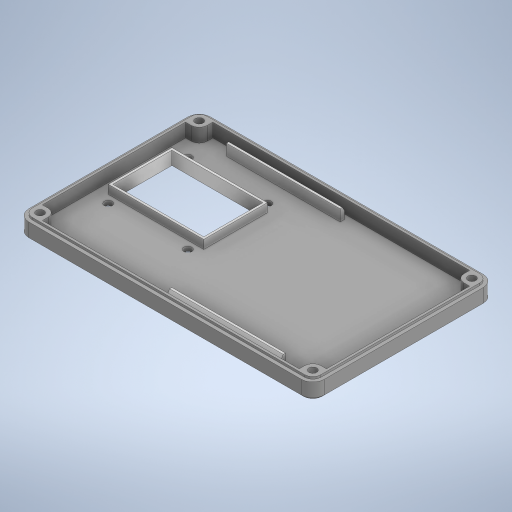
# Autodesk Inventor part: housing_top
Saved by Autodesk Inventor 2023 (Build 270158000, 158)
## iProperties
Created: 2023-05-16
Part Number: housing_top
Material: Generic
Document SubType Name: Modeling
Designer: mark
Density: 1 g/cm^3
Appearance: Default
Author: mark
Autodesk Inventor part; units mm, degrees
ref_plane "YZ Plane" through (0, 0, 0) normal (1, 0, 0) x (0, 1, 0)
ref_plane "XZ Plane" through (0, 0, 0) normal (0, 1, 0) x (-1, 0, 0)
ref_plane "XY Plane" through (0, 0, 0) normal (0, 0, 1) x (1, 0, 0)
sketch "Sketch1" plane through (0, 0, 0) normal (0, 1, 0) x (-1, 0, 0)
  line L0 (59.6914, -40.823) -> (-60.3086, -40.823)
  line L1 (-65.3086, -35.823) -> (-65.3086, 34.177)
  line L2 (-60.3086, 39.177) -> (59.6914, 39.177)
  line L3 (64.6914, 34.177) -> (64.6914, -35.823)
  arc A0 (59.6914, -40.823) -> (64.6914, -35.823) centre (59.6914, -35.823) ccw
  arc A1 (-65.3086, -35.823) -> (-60.3086, -40.823) centre (-60.3086, -35.823) ccw
  arc A2 (64.6914, 34.177) -> (59.6914, 39.177) centre (59.6914, 34.177) ccw
  arc A3 (-60.3086, 39.177) -> (-65.3086, 34.177) centre (-60.3086, 34.177) ccw
  point P0 (0, 0)
  point P1 (64.6914, -40.823)
  point P2 (-65.3086, 39.177)
  point P3 (64.6914, 39.177)
  dimension "d0" = 80
  dimension "d1" = 130
  dimension "d2" = 5
  dimension "d3" = 5
  dimension "d4" = 5
  dimension "d5" = 5
  constraints: 8 end point, 8 point on circle, 8 tangent, 6 point on line, 4 centre point, 2 parallel, 1 horizontal, 1 perpendicular
  measures "d0" distance of point (64.691, 39.177) point (64.691, -40.823)
  measures "d1" distance of point (-65.309, 39.177) point (64.691, 39.177)
  measures "d2" radius of A0
  measures "d3" radius of A1
  measures "d4" radius of A2
  measures "d5" radius of A3
extrude "Extrusion1" add sketch "Sketch1" along normal blind 2
sketch "Sketch2" plane through (0, 2, 0) normal (0, 1, 0) x (1, 0, 0)
  line L0 (-64.6914, 35.823) -> (-64.6914, -34.177) projected
  line L1 (-64.6914, 35.823) -> (-64.6914, -34.177)
  arc A0 (-64.6914, -34.177) -> (-59.6914, -39.177) centre (-59.6914, -34.177) ccw projected
  arc A1 (-64.6914, -34.177) -> (-59.6914, -39.177) centre (-59.6914, -34.177) ccw
  arc A2 (-59.6914, 40.823) -> (-64.6914, 35.823) centre (-59.6914, 35.823) ccw
  arc A3 (65.3086, 35.823) -> (60.3086, 40.823) centre (60.3086, 35.823) ccw projected
  arc A4 (65.3086, 35.823) -> (60.3086, 40.823) centre (60.3086, 35.823) ccw
  line L2 (-62.1914, 35.823) -> (-62.1914, -34.177)
  line L3 (65.3086, -34.177) -> (65.3086, 35.823) projected
  line L4 (65.3086, 35.823) -> (65.3086, -34.177)
  arc A5 (60.3086, -39.177) -> (65.3086, -34.177) centre (60.3086, -34.177) ccw projected
  line L5 (-59.6914, -39.177) -> (60.3086, -39.177) projected
  line L6 (60.3086, -39.177) -> (-59.6914, -39.177)
  line L7 (60.3086, 40.823) -> (-59.6914, 40.823) projected
  line L8 (-59.6914, 40.823) -> (60.3086, 40.823)
  line L9 (62.8086, 35.823) -> (62.8086, -34.177)
  line L10 (60.3086, -36.677) -> (-59.6914, -36.677)
  line L11 (-59.6914, 38.323) -> (60.3086, 38.323)
  arc A6 (-59.6914, 38.323) -> (-62.1914, 35.823) centre (-59.6914, 35.823) ccw
  arc A7 (62.8086, 35.823) -> (60.3086, 38.323) centre (60.3086, 35.823) ccw
  arc A8 (60.3086, -36.677) -> (62.8086, -34.177) centre (60.3086, -34.177) ccw
  arc A9 (-62.1914, -34.177) -> (-59.6914, -36.677) centre (-59.6914, -34.177) ccw
  arc A10 (-59.6914, 39.323) -> (-63.1914, 35.823) centre (-59.6914, 35.823) ccw
  arc A11 (63.8086, 35.823) -> (60.3086, 39.323) centre (60.3086, 35.823) ccw
  arc A12 (60.3086, -37.677) -> (63.8086, -34.177) centre (60.3086, -34.177) ccw
  arc A13 (-63.1914, -34.177) -> (-59.6914, -37.677) centre (-59.6914, -34.177) ccw
  line L12 (-63.1914, 35.823) -> (-63.1914, -34.177)
  line L13 (-59.6914, -37.677) -> (60.3086, -37.677)
  line L14 (63.8086, -34.177) -> (63.8086, 35.823)
  line L15 (60.3086, 39.323) -> (-59.6914, 39.323)
  line L16 (-59.6914, 32.323) -> (-62.1914, 32.323)
  line L17 (-56.1914, 35.823) -> (-56.1914, 38.323)
  arc A14 (-59.6914, 32.323) -> (-56.1914, 35.823) centre (-59.6914, 35.823) ccw
  line L18 (0.3086, 40.823) -> (0.3086, 33.323)
  line L19 (65.3086, 0.823) -> (44.6486, 0.823)
  line L20 (60.3086, 32.323) -> (62.8086, 32.323)
  line L21 (56.8086, 35.823) -> (56.8086, 38.323)
  arc A15 (56.8086, 35.823) -> (60.3086, 32.323) centre (60.3086, 35.823) ccw
  line L22 (-59.6914, -30.677) -> (-62.1914, -30.677)
  line L23 (-56.1914, -34.177) -> (-56.1914, -36.677)
  arc A16 (-56.1914, -34.177) -> (-59.6914, -30.677) centre (-59.6914, -34.177) ccw
  line L24 (56.8086, -34.177) -> (56.8086, -36.677)
  arc A17 (60.3086, -30.677) -> (56.8086, -34.177) centre (60.3086, -34.177) ccw
  line L25 (60.3086, -30.677) -> (62.8086, -30.677)
  point P0 (0, 0)
  point P1 (60.3086, -34.2192)
  point P2 (65.3086, -34.2192)
  point P3 (59.6599, -39.177)
  point P4 (56.8086, 38.323)
  point P5 (62.8086, -30.677)
  point P6 (56.8086, -36.677)
  point P7 (-56.1914, -36.677)
  point P8 (-62.1914, -30.677)
  dimension "d51" = 5
  dimension "d8" = 2.5
  dimension "d9" = 2.5
  dimension "d10" = 2.5
  dimension "d11" = 2.5
  dimension "d12" = 7
  dimension "d13" = 7
  dimension "d14" = 7
  dimension "d15" = 7
  dimension "d34" = 3.5
  dimension "d50" = 2.5
  dimension "d52" = 5
  dimension "d53" = 2.5
  constraints: 44 end point, 30 point on circle, 17 symmetric about line, 15 centre point, 11 coincident, 10 point on line, 10 tangent, 6 equal length, 3 vertical, 2 horizontal, 2 midpoint, 2 perpendicular, 7 other
  measures "d8" distance between parallel lines of L0 L2
  measures "d9" distance between parallel lines of L7 L11
  measures "d10" distance between parallel lines of L3 L9
  measures "d11" distance between parallel lines of L5 L10
  measures "d12" diameter of A10
  measures "d13" diameter of A11
  measures "d14" diameter of A12
  measures "d15" diameter of A13
  measures "d34" radius of A17
  measures "d50" radius of A8
  measures "d52" radius of A4
  measures "d53" radius of A7
extrude "Extrusion2" add sketch "Sketch2" along normal blind 5 contours A2 L7 L18 L15 A10 L12 A13 L13 A12 L14 L19 L3 A5 L5 A0 L0 | L7 A3 L3 L19 L14 A11 L15 L18 | L17 A14 L16 L2 A6 L11 | L11 A7 L9 L20 A15 L21 | L9 A8 L10 L24 A17 L25 | L22 A16 L23 L10 A9 L2
extrude "Extrusion3" add sketch "Sketch2" along normal blind 6 contours L18 L11 A6 L2 A9 L10 A8 L9 L19 L14 A12 L13 A13 L12 A10 L15 | L15 A11 L14 L19 L9 A7 L11 L18 | L17 A14 L16 L2 A6 L11 | L11 A7 L9 L20 A15 L21 | L9 A8 L10 L24 A17 L25 | L22 A16 L23 L10 A9 L2
sketch "Sketch3" plane through (0, 0, 0) normal (0, -1, 0) x (1, 0, 0)
  circle A0 centre (60.3086, 34.177) radius 3
  line L0 (-59.6914, 39.177) -> (60.3086, 39.177) projected
  line L1 (65.3086, 34.177) -> (65.3086, -35.823) projected
  line L2 (65.3086, 24.0261) -> (65.3086, 17.2129)
  line L3 (38.477, 39.177) -> (29.3328, 39.177)
  line L4 (-59.6914, 39.177) -> (60.3086, 39.177) projected
  circle A1 centre (60.3086, -35.823) radius 3
  circle A2 centre (-59.6914, 34.177) radius 3
  circle A3 centre (-59.6914, -35.823) radius 3
  line L5 (-64.6914, -35.823) -> (-64.6914, 34.177) projected
  line L6 (60.3086, -40.823) -> (-59.6914, -40.823) projected
  point P0 (0, 0)
  point P1 (33.602, 39.1426)
  point P2 (55.3086, 34.177)
  point P3 (65.3086, -35.823)
  dimension "d20" = 6
  dimension "d21" = 5
  dimension "d26" = 70
  dimension "d29" = 120
  dimension "d54" = 130
  dimension "d55" = 80
  dimension "d56" = 5
  constraints: 4 centre point, 4 end point, 2 point on line, 1 equal radius, 1 horizontal, 1 vertical alignment, 7 other
  measures "d20" diameter of A0
  measures "d21" distance from line of L0 A0.centre
  measures "d26" distance of A0.centre A1.centre
  measures "d29" distance of A0.centre A2.centre
  measures "d55" distance between parallel lines of L0 L6
extrude "Extrusion4" cut sketch "Sketch3" against normal blind 3
sketch "Sketch4" plane through (60.3086, 3, -35.823) normal (0, -1, 0) x (1, 0, 0)
  circle A0 centre (0, 0) radius 3 projected
  point P0 (-60.3086, 35.823)
  constraints: 1 coincident
hole "Hole1" at (60.3086, 3, -35.823) direction (0, 1, 0) diameter 3.5 end through all
pattern_linear "Rectangular Pattern1" count 2 spacing 120 along (-1, 0, 0) count 2 spacing 70 along (0, 0, 1) of "Hole1"
chamfer "Chamfer1" distance 1 angle 45 8 edges at (0.3086, 0, 39.177) (63.8442, 0, 37.7125) (65.3086, 0, -0.823) (63.8442, 0, -39.3586) (0.3086, 0, -40.823) (-63.2269, 0, -39.3586) (-64.6914, 0, -0.823) (-63.2269, 0, 37.7125)
sketch "Sketch9" plane through (0, 0, 0) normal (0, -1, 0) x (1, 0, 0)
  line L0 (-8.8254, 34.5739) -> (9.2353, 34.5739) construction
  line L1 (9.2353, 34.5739) -> (9.2353, 29.7737) construction
  line L2 (9.2353, 29.7737) -> (-8.8254, 29.7737) construction
  line L3 (-8.8254, 29.7737) -> (-8.8254, 34.5739) construction
  point P0 (0, 0)
  constraints: 2 other
sketch "Sketch10" plane through (0, 2, 0) normal (0, 1, 0) x (1, 0, 0)
  line L0 (46.8086, -34.677) -> (-3.1914, -34.677)
  line L1 (-3.1914, -34.677) -> (-3.1914, -32.677)
  line L2 (-3.1914, -32.677) -> (46.8086, -32.677)
  line L3 (46.8086, -32.677) -> (46.8086, -34.677)
  line L4 (56.8086, -34.177) -> (56.8086, -36.677) projected
  line L5 (56.8086, -36.677) -> (-56.1914, -36.677) projected
  line L6 (-46.1914, 36.323) -> (3.8086, 36.323)
  line L7 (3.8086, 36.323) -> (3.8086, 34.323)
  line L8 (3.8086, 34.323) -> (-46.1914, 34.323)
  line L9 (-46.1914, 34.323) -> (-46.1914, 36.323)
  line L10 (-56.1914, 38.323) -> (56.8086, 38.323) projected
  line L11 (-56.1914, 35.823) -> (-56.1914, 38.323) projected
  point P0 (0, 0)
  point P1 (56.8086, -35.427)
  point P2 (46.8086, -33.677)
  point P3 (-3.1914, -36.677)
  point P4 (-46.1914, 35.323)
  point P5 (-56.1914, 37.073)
  dimension "d97" = 50
  dimension "d98" = 2
  dimension "d99" = 10
  dimension "d100" = 2
  dimension "d110" = 50
  dimension "d111" = 2
  dimension "d112" = 2
  dimension "d113" = 10
  constraints: 16 end point, 4 midpoint, 4 parallel, 2 horizontal, 2 perpendicular, 1 point on line
  measures "d97" distance of L1.end L2.end
  measures "d98" distance of L0.end L1.end
  measures "d99" horizontal distance of point (56.809, -35.427) point (46.809, -33.677)
  measures "d100" distance between parallel lines of L5 L0
  measures "d110" distance of L7.end L8.end
  measures "d111" distance of L6.end L7.end
  measures "d112" distance between parallel lines of L10 L6
  measures "d113" horizontal distance of point (-46.191, 35.323) point (-56.191, 37.073)
extrude "Extrusion7" add sketch "Sketch10" along normal blind 5
chamfer "Chamfer2" distance 1 angle 60 1 edges at (21.8086, 7, 34.677) measured on face at (13.4753, 7, 33.3436)
chamfer "Chamfer4" distance 1 angle 60 1 edges at (-21.1914, 7, -36.323) measured on face at (-29.5247, 7, -35.6564)
sketch "Sketch11" plane through (0, 0, 0) normal (0, -1, 0) x (1, 0, 0)
  line L0 (-56.6914, 5.177) -> (-16.6914, 5.177)
  line L1 (-16.6914, 5.177) -> (-16.6914, -20.823)
  line L2 (-16.6914, -20.823) -> (-56.6914, -20.823)
  line L3 (-56.6914, -20.823) -> (-56.6914, 5.177)
  line L4 (-64.6914, 34.177) -> (-64.6914, -35.823) projected
  line L5 (-59.6914, -40.823) -> (60.3086, -40.823) projected
  point P0 (0, 0)
  dimension "d117" = 40
  dimension "d118" = 26
  dimension "d119" = 8
  dimension "d120" = 20
  constraints: 8 end point, 2 parallel, 1 horizontal, 1 perpendicular
  measures "d117" distance of L1.end L2.end
  measures "d118" distance of L0.end L1.end
  measures "d119" distance between parallel lines of L4 L3
  measures "d120" distance between parallel lines of L5 L2
extrude "Extrusion8" cut sketch "Sketch11" against normal blind 10
sketch "Sketch12" plane through (0, 2, 0) normal (0, 1, 0) x (1, 0, 0)
  line L0 (-57.6914, 28.823) -> (-15.6914, 28.823)
  line L1 (-15.6914, 28.823) -> (-15.6914, -13.177)
  line L2 (-15.6914, -13.177) -> (-57.6914, -13.177)
  line L3 (-57.6914, -13.177) -> (-57.6914, 28.823)
  line L4 (-16.6914, -5.177) -> (-56.6914, -5.177) projected
  line L5 (-16.6914, 20.823) -> (-16.6914, -5.177) projected
  circle A0 centre (-54.1914, 25.323) radius 1.75
  circle A1 centre (-19.1914, 25.323) radius 1.75
  circle A2 centre (-54.1914, -9.677) radius 1.75
  circle A3 centre (-19.1914, -9.677) radius 1.75
  point P0 (0, 0)
  dimension "d127" = 42
  dimension "d128" = 42
  dimension "d129" = 8
  dimension "d130" = 1
  dimension "d131" = 3.5
  dimension "d132" = 3.5
  dimension "d133" = 3.5
  dimension "d136" = 35
  dimension "d139" = 35
  constraints: 8 end point, 4 centre point, 2 horizontal, 2 parallel, 1 perpendicular, 1 vertical, 6 other
  measures "d127" distance of L1.end L2.end
  measures "d128" distance of L0.end L1.end
  measures "d129" distance between parallel lines of L2 L4
  measures "d130" distance between parallel lines of L1 L5
  measures "d131" diameter of A0
  measures "d132" distance from line of L0 A0.centre
  measures "d133" distance from line of A0.centre L3
  measures "d136" distance of A0.centre A1.centre
  measures "d139" distance of A0.centre A2.centre
extrude "Extrusion9" cut sketch "Sketch12" against normal blind 10 contours A0 | A1 | A2 | A3
sketch "Sketch13" plane through (0, 2, 0) normal (0, 1, 0) x (1, 0, 0)
  line L0 (-57.6914, -6.177) -> (-15.6914, -6.177)
  line L1 (-15.6914, -6.177) -> (-15.6914, 21.823)
  line L2 (-15.6914, 21.823) -> (-57.6914, 21.823)
  line L3 (-57.6914, 21.823) -> (-57.6914, -6.177)
  line L4 (-56.6914, 20.823) -> (-16.6914, 20.823) projected
  line L5 (-56.6914, -5.177) -> (-16.6914, -5.177)
  line L6 (-16.6914, -5.177) -> (-16.6914, 20.823)
  line L7 (-16.6914, 20.823) -> (-56.6914, 20.823)
  line L8 (-56.6914, 20.823) -> (-56.6914, -5.177)
  point P0 (0, 0)
  dimension "d144" = 1
  dimension "d145" = 1
  dimension "d146" = 1
  dimension "d147" = 1
  constraints: 16 end point, 4 parallel, 2 horizontal, 2 perpendicular
  measures "d144" distance between parallel lines of L8 L3
  measures "d145" distance between parallel lines of L5 L0
  measures "d146" distance between parallel lines of L4 L2
  measures "d147" distance between parallel lines of L6 L1
extrude "Extrusion10" add sketch "Sketch13" along normal blind 3.8
equation "\"d3\" = d2"
equation "\"d4\" = d2"
equation "\"d5\" = d2"
equation "\"d9\" = d8"
equation "\"d10\" = d8"
equation "\"d11\" = d8"
equation "\"d52\" = d51"
equation "\"d53\" = d50"
body "Solid1"
